y_endstop_holder (Autodesk Fusion 360 design; units mm, degrees)
Autodesk Fusion 360 part; units mm, degrees
note: some values were not read from the file. Chosen so that the rebuilt part matches the saved one: where a step starts.
sketch "Sketch1" plane through (0, 0, 0) normal (1, 0, 0) x (0, 0, -1)
  line L0 (-7, 3.8) -> (-3.995, 3.8)
  line L1 (3.995, 3.8) -> (7, 3.8)
  line L2 (7, 3.8) -> (7, 10.3)
  line L3 (7, 10.3) -> (14, 10.3)
  line L4 (14, 10.3) -> (14, -1.7)
  line L5 (14, -1.7) -> (4, -9.7)
  line L6 (4, -9.7) -> (-4, -9.7)
  line L7 (-4, -9.7) -> (-14, -1.7)
  line L8 (-14, -1.7) -> (-14, 10.3)
  line L9 (-7, 10.3) -> (-7, 3.8)
  line L10 (-7, 10.3) -> (-14, 10.3)
  arc A0 (-3.4641, 2) -> (3.4641, 2) centre (0, 0) ccw
  arc A1 (-3.995, 3.8) -> (-3.4641, 2) centre (0, 4) ccw
  arc A2 (3.4641, 2) -> (3.995, 3.8) centre (0, 4) ccw
  point P0 (0, -9.7)
  dimension "d1" = 8
  dimension "d2" = 28
  dimension "d3" = 14
  dimension "d4" = 14
  dimension "d5" = 7
  dimension "d6" = 6.5
  dimension "d7" = 20
  dimension "d8" = 12
  dimension "d9" = 8
  dimension "d10" = 0.2
  constraint coincident A0.centre origin
  constraint coincident A1.centre A0
  constraint equal A0 A1
  constraint vertical A0.centre A1.centre
  constraint horizontal L0
  constraint parallel L0 L1
  constraint perpendicular L1 L2
  constraint perpendicular L2 L3
  constraint perpendicular L3 L4
  constraint perpendicular L4 L6
  constraint parallel L4 L8
  constraint perpendicular L8 L10
  constraint vertical L9
  constraint collinear L3 L10
  constraint collinear L0 L1
  constraint coincident A0.end A1
  constraint concentric A1 A2
  constraint midpoint L6 P0
  constraint vertical A0.centre P0
  constraint horizontal L4.end L7.end
  measures "d1" diameter of A1
  measures "d2" distance of L4 L8
  measures "d3" distance of A1.centre L8
  measures "d4" distance of L2 L9
  measures "d5" horizontal distance of A1.centre L0.start
  measures "d6" distance of L0.start L9.start
  measures "d7" distance of L6 L10
  measures "d8" distance of L7.end L8.end
  measures "d9" distance of L5.end L6.end
  measures "d10" distance of L0 A1.centre
extrude "Extrude1" add sketch "Sketch1" along normal blind 6
sketch "Sketch2" plane through (0, 10.3, 0) normal (0, 1, 0) x (-1, 0, 0)
  line L0 (0, 7) -> (0, 14)
  line L1 (0, 14) -> (-6, 14)
  line L2 (-6, 14) -> (-6, 7)
  line L3 (-6, 7) -> (0, 7)
  circle A0 centre (-3, -9.5) radius 2
  circle A1 centre (-3, 9.5) radius 2
  circle A2 centre (-3, -9.5) radius 1.6
  circle A3 centre (-3, 9.5) radius 1.6
  point P0 (-3, 14)
  dimension "d13" = 4
  dimension "d14" = 19
  dimension "d15" = 9.5
  dimension "d16" = 3.2
  constraint midpoint L1 P0
  constraint vertical A1.centre P0
  constraint vertical A0.centre A1.centre
  constraint equal A0 A1
  constraint concentric A0 A2
  constraint concentric A1 A3
  constraint equal A2 A3
  measures "d13" diameter of A0
  measures "d14" distance of A0.centre A1.centre
  measures "d15" vertical distance of origin A1.centre
  measures "d16" diameter of A3
extrude "Extrude2" cut sketch "Sketch2" against normal through all contours A2 | A3
extrude "Extrude3" cut sketch "Sketch2" against normal blind 12 from surface at -6.5 contours A0 | A1
extrude "Extrude4" cut 2 faces at (2.9601, 10.3, 13.0318) (2.9601, 10.3, -13.0318) along direction (0, -1, 0) through all from surface at 7 start surface through (0, 3.8, 0) normal (0, -1, 0)
equation "d3 = d2 / 2"
equation "d5 = d4 / 2"
equation "d15 = d14 / 2"
